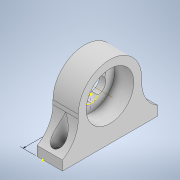
# Autodesk Inventor part: Motor Mount V1
Saved by Autodesk Inventor 2020 (Build 240168000, 168)
## iProperties
Created: 2020-01-13
Part Number: Motor Mount V1
Material: Generic
Document SubType Name: Modeling
Designer: maple
Density: 1 g/cm^3
Appearance: Default
Author: maple
Autodesk Inventor part; units mm, degrees
ref_plane "YZ Plane" through (0, 0, 0) normal (1, 0, 0) x (0, 1, 0)
ref_plane "XZ Plane" through (0, 0, 0) normal (0, 1, 0) x (-1, 0, 0)
ref_plane "XY Plane" through (0, 0, 0) normal (0, 0, 1) x (1, 0, 0)
sketch "Sketch1" plane through (0, 0, 0) normal (0, 1, 0) x (-1, 0, 0)
  line L0 (0, 0) -> (-20.32, 0)
  line L1 (-20.32, 0) -> (-20.32, -76.2)
  line L2 (-20.32, -76.2) -> (0, -76.2)
  line L3 (0, -76.2) -> (0, 0)
  dimension "d0" = 20.32
  dimension "d1" = 76.2
  constraints: 8 end point, 2 parallel, 1 horizontal, 1 perpendicular
  measures "d0" distance of L2.end L1.end
  measures "d1" distance of L1.end L0.end
extrude "Extrusion1" add sketch "Sketch1" along normal blind 7.62
sketch "Sketch2" plane through (0, 7.62, 0) normal (0, 1, 0) x (1, 0, 0)
  line L0 (0, 0) -> (0, 12.7)
  line L1 (0, 76.2) -> (0, 0) projected
  line L2 (20.32, 0) -> (20.32, 76.2) projected
  line L3 (0, 12.7) -> (20.32, 12.7)
  line L4 (20.32, 12.7) -> (20.32, 63.5)
  line L5 (20.32, 63.5) -> (0, 63.5)
  line L6 (0, 63.5) -> (0, 12.7)
  dimension "d4" = 12.7
  dimension "d5" = 50.8
  constraints: 10 end point, 2 parallel, 2 point on line, 1 horizontal, 1 perpendicular
  measures "d4" distance of L0.start L0.end
  measures "d5" distance of L4.end L3.end
extrude "Extrusion2" add sketch "Sketch2" along normal blind 50.8
sketch "Sketch3" plane through (20.32, 0, 0) normal (1, 0, 0) x (0, 0, -1)
  line L0 (12.7, 58.42) -> (63.5, 58.42) projected
  line L1 (38.1, 58.42) -> (38.1, 33.02)
  circle A0 centre (38.1, 33.02) radius 19.05
  point P0 (0, 0)
  dimension "d8" = 25.4
  dimension "d9" = 38.1
  constraints: 2 end point, 1 centre point, 1 coincident, 1 midpoint, 1 vertical
  measures "d8" distance of L1.start L1.end
  measures "d9" diameter of A0
extrude "Extrusion3" cut sketch "Sketch3" against normal blind 15.24
sketch "Sketch4" plane through (5.08, 33.02, -38.1) normal (1, 0, 0) x (0, 0, -1)
  circle A0 centre (0, 0) radius 19.05 projected
  line L0 (0, 19.05) -> (0, 12.7)
  line L1 (0, 12.7) -> (0, 6.35)
  circle A1 centre (0, 6.35) radius 6.35
  point P0 (-38.1, -33.02)
  dimension "d12" = 6.35
  dimension "d13" = 6.35
  dimension "d14" = 12.7
  constraints: 4 end point, 2 vertical, 1 centre point, 1 coincident, 1 vertical alignment, 1 other
  measures "d12" distance of L0.start L0.end
  measures "d13" distance of L0.end L1.end
  measures "d14" diameter of A1
extrude "Extrusion4" cut sketch "Sketch4" against normal blind 5.08 contours A1
sketch "Sketch5" plane through (5.08, 33.02, -38.1) normal (1, 0, 0) x (0, 0, -1)
  circle A0 centre (0, 6.35) radius 6.35 projected
  point P0 (-38.1, -33.02)
  point P1 (0, 0)
  constraints: 1 vertical alignment, 1 other
pattern_circular "Circular Pattern1" count 6 over 360 about axis through (5.08, 33.02, -38.1) along (1, 0, 0) of "Extrusion4"
fillet "Fillet1" radius 25.4 1 edges at (10.16, 58.42, -12.7)
fillet "Fillet2" radius 25.4 1 edges at (10.16, 58.42, -63.5)
sketch "Sketch6" plane through (0, 7.62, 0) normal (0, 1, 0) x (1, 0, 0)
  line L0 (0, 12.7) -> (20.32, 12.7) projected
  line L1 (10.16, 12.7) -> (10.16, 2.54)
  line L2 (10.16, 12.7) -> (10.16, 7.62)
  line L3 (0, 63.5) -> (20.32, 63.5) projected
  line L4 (10.16, 63.5) -> (10.16, 68.58)
  circle A0 centre (10.16, 7.62) radius 2.54
  circle A1 centre (10.16, 68.58) radius 2.54
  point P0 (0, 0)
  dimension "d24" = 10.16
  dimension "d25" = 5.08
  dimension "d26" = 5.08
  dimension "d27" = 5.08
  dimension "d28" = 5.08
  constraints: 6 end point, 3 midpoint, 2 centre point, 2 coincident, 2 vertical
  measures "d24" distance of L1.start L1.end
  measures "d25" distance of L1.start L2.end
  measures "d26" distance of L4.start L4.end
  measures "d27" diameter of A0
  measures "d28" diameter of A1
fillet "Fillet5" radius 25.4 2 edges at (10.16, 7.62, -63.5) (10.16, 7.62, -12.7)
hole "Hole1" at (10.16, 7.62, -7.62) at (10.16, 7.62, -68.58) direction (0, -1, 0) diameter 5.08 end through all counterbore diameter 10.16 counterbore depth 3.81
sketch "Sketch8" plane through (10.16, 7.62, -7.62) normal (0, -1, 0) x (1, 0, 0)
  circle A0 centre (0, 0) radius 5.08
  circle A1 centre (0, -60.96) radius 2.54 projected
  line L0 (-2.54, -60.96) -> (0, -60.96)
  circle A2 centre (0, -60.96) radius 5.08
  point P0 (-10.16, 7.62)
  dimension "d37" = 10.16
  dimension "d38" = 10.16
  constraints: 2 centre point, 2 end point, 1 coincident, 1 horizontal, 1 horizontal alignment, 1 other
  measures "d37" diameter of A0
  measures "d38" diameter of A2
extrude "Extrusion5" cut sketch "Sketch8" against normal blind 25.4 contours A0 | A1 | A2
sketch "Sketch9" plane through (5.08, 33.02, -38.1) normal (1, 0, 0) x (0, 0, -1)
  arc A0 (5.4993, 9.525) -> (-5.4993, 9.525) centre (0, 6.35) ccw projected
  arc A1 (-5.4993, -9.525) -> (5.4993, -9.525) centre (0, -6.35) ccw projected
  point P0 (-38.1, -33.02)
  point P1 (0, 12.7)
  point P2 (0, -12.7)
  constraints: 2 point on circle
body "Solid1"
